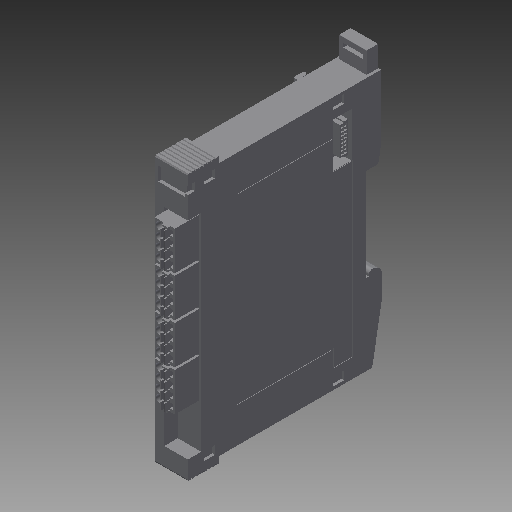
# Autodesk Inventor part: 178772
Saved by Autodesk Inventor 2019.3 (Build 233278000, 278)
## iProperties
Category: PARTsolutions
Company: MOELLER
Created: 2018-10-25
Part Number: 178772
Material: Generic
Catalog Web Link: www.cadenas.de
Description: I/O Modules-
Vendor: MOELLER
Document SubType Name: Modeling
Designer: psadmin
Manufacturer: MOELLER
Mass: 87.1869 g
Surface Area: 238.009 cm^2
Volume: 87.1869 cm^3
Density: 1 g/cm^3
Appearance: PSOLRGB-175-175-175
PSOL_IDENT_0: {$CADENAS_DATA\23d-libs\moeller\1589\1737\1739\1743\1744.prj},170 {VTYP=3D},{NB=178772},{LINA=178772
PSOL_IDENT_1: },{NN=I/O Modules},{DATE=04.10.2018 12:16:38},{GEOMDATE=04.10.2018 08:29:25},{VERSION=v181004082925}
PSOL_IDENT_2: ,{LINEID=10},{WBVAR=},{WBNUMERIC=}  {NB=178772},{LINA=178772},{KT=DUMMY},{PFOTO=2723pic-251.jpg},{PL
PSOL_IDENT_3: ID=178772},{DATA_SHEET=Data sheet},{MANUTYPEDESC=XN-322-4AI-PTNI},{DESCSHORT=Analog input module; 4
PSOL_IDENT_4: analog inputs; Pt/Ni/KTY/R with 2-wire or 3-wire connection},{DESCLONG=Analog input module for four
PSOL_IDENT_5: Pt100/Pt1000/Ni100/Ni1000/KTYxx/R resistance inputs with 2-wire and 3-wire configurations},{EAN=7640
PSOL_IDENT_6: 130098367},{ECLASS_8_1=27-24-26-01},{PACKAGED_WEIGHT=0.056},{DATA_SHEET_=http://datasheet.moeller.ne
PSOL_IDENT_7: t/datasheet.php?model=178772&locale=en_GB},{DATA_SHEET_ENG=http://datasheet.moeller.net/datasheet.ph
PSOL_IDENT_8: p?model=178772&locale=en_GB},{DATA_SHEET_DEU=http://datasheet.moeller.net/datasheet.php?model=178772
PSOL_IDENT_9: &locale=de_DE}
NN: I/O Modules
NB: 178772
NBSYN: $PLID.
LINA: 178772
PFOTO: 2723pic-251.jpg
PLID: 178772
DATA_SHEET: Data sheet
MANUTYPEDESC: XN-322-4AI-PTNI
DESCSHORT: Analog input module; 4 analog inputs; Pt/Ni/KTY/R with 2-wire or 3-wire connection
DESCLONG: Analog input module for four Pt100/Pt1000/Ni100/Ni1000/KTYxx/R resistance inputs with 2-wire and 3-wire configurations
EAN: 7640130098367
ECLASS_8_1: 27-24-26-01
PACKAGED_WEIGHT: 0.056
SUPPLIER: MOELLER
ARTICLENO: 178772
BOMINFO: 178772
CREATOR: CADENAS GmbH
Title: 178772
Author: Cadenas PARTsolutions
Autodesk Inventor part; units mm, degrees
(part 1 of 2)
ref_plane "YZ Plane" through (0, 0, 0) normal (1, 0, 0) x (0, 1, 0)
ref_plane "XZ Plane" through (0, 0, 0) normal (0, 1, 0) x (-1, 0, 0)
ref_plane "XY Plane" through (0, 0, 0) normal (0, 0, 1) x (1, 0, 0)
sketch "Sketch_31" plane through (0, 0, 0) normal (1, 0, 0) x (0, 1, 0)
  line L0 (50.4, 37) -> (-50.4, 37)
  line L1 (-50.4, 37) -> (-50.9, 36.75)
  line L2 (-50.9, 36.75) -> (-50.9, 35.75)
  line L3 (-50.9, 35.75) -> (-50.4, 35.5)
  line L4 (-50.4, 35.5) -> (-50.9, 35.25)
  line L5 (-50.9, 35.25) -> (-50.9, 34.25)
  line L6 (-50.9, 34.25) -> (-50.4, 34)
  line L7 (-50.4, 34) -> (-50.9, 33.75)
  line L8 (-50.9, 33.75) -> (-50.9, 32.75)
  line L9 (-50.9, 32.75) -> (-50.4, 32.5)
  line L10 (-50.4, 32.5) -> (-50.9, 32.25)
  line L11 (-50.9, 32.25) -> (-50.9, 31.25)
  line L12 (-50.9, 31.25) -> (-50.4, 31)
  line L13 (-50.4, 31) -> (-50.9, 30.75)
  line L14 (-50.9, 30.75) -> (-50.9, 29.75)
  line L15 (-50.9, 29.75) -> (-50.4, 29.5)
  line L16 (-50.4, 29.5) -> (-50.9, 29.25)
  line L17 (-50.9, 29.25) -> (-50.9, 28.25)
  line L18 (-50.9, 28.25) -> (-50.4, 28)
  line L19 (-50.4, 28) -> (-50.9, 27.75)
  line L20 (-50.9, 27.75) -> (-50.9, 26.75)
  line L21 (-50.9, 26.75) -> (-50.4, 26.5)
  line L22 (-50.4, 26.5) -> (-50.9, 26.25)
  line L23 (-50.9, 26.25) -> (-50.9, 25.25)
  line L24 (-50.9, 25.25) -> (-50.4, 25)
  line L25 (-50.4, 25) -> (-48.5, 25)
  line L26 (-48.5, 25) -> (-48.5, -32.7457)
  arc A0 (-48.5, -32.7457) -> (-47.6723, -33.7308) centre (-47.5, -32.7457) ccw
  line L27 (-47.6723, -33.7308) -> (-28.35, -37.11)
  line L28 (-28.35, -37.11) -> (-18.1454, -37.11)
  arc A1 (-18.1454, -37.11) -> (-17.2257, -36.6632) centre (-18.1454, -35.94) ccw
  line L29 (-17.2257, -36.6632) -> (-16.339, -35.5357)
  arc A2 (-16.339, -35.5357) -> (-16.3079, -35.4792) centre (-16.4962, -35.4121) ccw
  line L30 (-16.3079, -35.4792) -> (-15.785, -34.013)
  arc A3 (-15.785, -34.013) -> (-16.2215, -32.6577) centre (-16.887, -33.62) ccw
  line L31 (-16.2215, -32.6577) -> (-16.3517, -32.5677)
  arc A4 (-16.3517, -32.5677) -> (-17.0171, -32.36) centre (-17.0171, -33.53) ccw
  line L32 (-17.0171, -32.36) -> (-17.727, -32.36)
  line L33 (-17.727, -32.36) -> (-17.727, -31.25)
  line L34 (-17.727, -31.25) -> (17.833, -31.25)
  line L35 (17.833, -31.25) -> (17.833, -35.1079)
  arc A5 (17.833, -35.1079) -> (18.6743, -36.0952) centre (18.833, -35.1079) ccw
  line L36 (18.6743, -36.0952) -> (24.303, -37)
  line L37 (24.303, -37) -> (48.56, -37)
  line L38 (48.56, -37) -> (48.56, 25)
  line L39 (48.56, 25) -> (50.4, 25)
  line L40 (50.4, 25) -> (50.9, 25.25)
  line L41 (50.9, 25.25) -> (50.9, 26.25)
  line L42 (50.9, 26.25) -> (50.4, 26.5)
  line L43 (50.4, 26.5) -> (50.9, 26.75)
  line L44 (50.9, 26.75) -> (50.9, 27.75)
  line L45 (50.9, 27.75) -> (50.4, 28)
  line L46 (50.4, 28) -> (50.9, 28.25)
  line L47 (50.9, 28.25) -> (50.9, 29.25)
  line L48 (50.9, 29.25) -> (50.4, 29.5)
  line L49 (50.4, 29.5) -> (50.9, 29.75)
  line L50 (50.9, 29.75) -> (50.9, 30.75)
  line L51 (50.9, 30.75) -> (50.4, 31)
  line L52 (50.4, 31) -> (50.9, 31.25)
  line L53 (50.9, 31.25) -> (50.9, 32.25)
  line L54 (50.9, 32.25) -> (50.4, 32.5)
  line L55 (50.4, 32.5) -> (50.9, 32.75)
  line L56 (50.9, 32.75) -> (50.9, 33.75)
  line L57 (50.9, 33.75) -> (50.4, 34)
  line L58 (50.4, 34) -> (50.9, 34.25)
  line L59 (50.9, 34.25) -> (50.9, 35.25)
  line L60 (50.9, 35.25) -> (50.4, 35.5)
  line L61 (50.4, 35.5) -> (50.9, 35.75)
  line L62 (50.9, 35.75) -> (50.9, 36.75)
  line L63 (50.9, 36.75) -> (50.4, 37)
  constraints: 128 end point, 12 point on circle, 6 centre point
extrude "Extrusion1" add sketch "Sketch_31" along normal mid plane 12.5
sketch "Sketch_3" plane through (0, 0, 35.91) normal (0, 0, 1) x (1, 0, 0)
  line L0 (-2.75, 35.485) -> (-2.75, -43.665)
  line L1 (-2.75, -43.665) -> (6.25, -43.665)
  line L2 (6.25, -43.665) -> (6.25, 35.485)
  line L3 (6.25, 35.485) -> (-2.75, 35.485)
  constraints: 8 end point
extrude "Extrusion2" cut sketch "Sketch_3" along normal mid plane 8.12
sketch "Sketch_4" plane through (0, -4.03, 35.91) normal (0, 1, 0) x (1, 0, 0)
  line L0 (-2.242, 6.138) -> (-2.242, -5.332)
  line L1 (-2.242, -5.332) -> (5.508, -5.332)
  line L2 (5.508, -5.332) -> (5.508, 6.138)
  line L3 (5.508, 6.138) -> (-2.242, 6.138)
  constraints: 8 end point
extrude "Extrusion3" add sketch "Sketch_4" along normal mid plane 77.15
sketch "Sketch_7" plane through (0, 0, 35.91) normal (0, 0, 1) x (1, 0, 0)
  line L0 (-5.1, 48.02) -> (-5.1, 42.82)
  line L1 (-5.1, 42.82) -> (5.1, 42.82)
  line L2 (5.1, 42.82) -> (5.1, 43.92)
  line L3 (5.1, 43.92) -> (7.9, 43.92)
  line L4 (7.9, 43.92) -> (7.9, 46.92)
  line L5 (7.9, 46.92) -> (5.1, 46.92)
  line L6 (5.1, 46.92) -> (5.1, 48.02)
  line L7 (5.1, 48.02) -> (-5.1, 48.02)
  constraints: 16 end point
extrude "Extrusion4" cut sketch "Sketch_7" along normal mid plane 3.2
sketch "Sketch_8" plane through (0, 0, 35.91) normal (0, 0, 1) x (1, 0, 0)
  line L0 (-5, 47.92) -> (-5, 42.92)
  line L1 (-5, 42.92) -> (5, 42.92)
  line L2 (5, 42.92) -> (5, 47.92)
  line L3 (5, 47.92) -> (-5, 47.92)
  constraints: 8 end point
extrude "Extrusion5" add sketch "Sketch_8" against normal blind 2
sketch "Sketch_20" plane through (0, 0, 41.242) normal (0, 0, 1) x (1, 0, 0)
  line L0 (-2.165, -42.605) -> (2.835, -42.605)
  line L1 (2.835, -42.605) -> (2.835, 34.545)
  line L2 (2.835, 34.545) -> (-2.165, 34.545)
  line L3 (-2.165, 34.545) -> (-2.165, -42.605)
  constraints: 8 end point
sketch "Sketch_21" plane through (0, 0, 41.242) normal (0, 0, 1) x (1, 0, 0)
  line L0 (-2.165, -42.605) -> (2.835, -42.605)
  line L1 (2.835, -42.605) -> (2.835, 34.545)
  line L2 (2.835, 34.545) -> (-2.165, 34.545)
  line L3 (-2.165, 34.545) -> (-2.165, -42.605)
  circle A0 centre (-0.2, 32.542) radius 1.5
  circle A1 centre (-0.2, 29.042) radius 1.5
  circle A2 centre (-0.2, 25.542) radius 1.5
  circle A3 centre (-0.2, 22.042) radius 1.5
  circle A4 centre (-0.2, 16.942) radius 1.5
  circle A5 centre (-0.2, 13.442) radius 1.5
  circle A6 centre (-0.2, 9.942) radius 1.5
  circle A7 centre (-0.2, 6.442) radius 1.5
  circle A8 centre (-0.2, 1.342) radius 1.5
  circle A9 centre (-0.2, -2.158) radius 1.5
  circle A10 centre (-0.2, -5.658) radius 1.5
  circle A11 centre (-0.2, -9.158) radius 1.5
  circle A12 centre (-0.2, -14.258) radius 1.5
  circle A13 centre (-0.2, -17.758) radius 1.5
  circle A14 centre (-0.2, -21.258) radius 1.5
  circle A15 centre (-0.2, -24.758) radius 1.5
  circle A16 centre (-0.2, -29.858) radius 1.5
  circle A17 centre (-0.2, -33.358) radius 1.5
  circle A18 centre (-0.2, -36.858) radius 1.5
  circle A19 centre (-0.2, -40.358) radius 1.5
  constraints: 20 centre point, 8 end point
extrude "Extrusion6" cut sketch "Sketch_20" along normal mid plane 6.6
extrude "Extrusion7" add sketch "Sketch_21" against normal blind 3.3
sketch "Sketch_10" plane through (0, 0, 41.242) normal (0, 0, 1) x (1, 0, 0)
  line L0 (1.508, -42.605) -> (5.508, -42.605)
  line L1 (5.508, -42.605) -> (5.508, 34.545)
  line L2 (5.508, 34.545) -> (1.508, 34.545)
  line L3 (1.508, 34.545) -> (1.508, -42.605)
  constraints: 8 end point
sketch "Sketch_11" plane through (0, 0, 41.242) normal (0, 0, 1) x (1, 0, 0)
  line L0 (1.508, -42.605) -> (5.508, -42.605)
  line L1 (5.508, -42.605) -> (5.508, 34.545)
  line L2 (5.508, 34.545) -> (1.508, 34.545)
  line L3 (1.508, 34.545) -> (1.508, -42.605)
  line L4 (3.55, 31.392) -> (4.6, 31.392)
  arc A0 (4.6, 31.392) -> (4.9, 31.692) centre (4.6, 31.692) ccw
  line L5 (4.9, 31.692) -> (4.9, 33.142)
  arc A1 (4.9, 33.142) -> (4.6, 33.442) centre (4.6, 33.142) ccw
  line L6 (4.6, 33.442) -> (3.55, 33.442)
  line L7 (3.55, 33.442) -> (3.55, 31.392)
  line L8 (3.55, 27.892) -> (4.6, 27.892)
  arc A2 (4.6, 27.892) -> (4.9, 28.192) centre (4.6, 28.192) ccw
  line L9 (4.9, 28.192) -> (4.9, 29.642)
  arc A3 (4.9, 29.642) -> (4.6, 29.942) centre (4.6, 29.642) ccw
  line L10 (4.6, 29.942) -> (3.55, 29.942)
  line L11 (3.55, 29.942) -> (3.55, 27.892)
  line L12 (3.55, 24.392) -> (4.6, 24.392)
  arc A4 (4.6, 24.392) -> (4.9, 24.692) centre (4.6, 24.692) ccw
  line L13 (4.9, 24.692) -> (4.9, 26.142)
  arc A5 (4.9, 26.142) -> (4.6, 26.442) centre (4.6, 26.142) ccw
  line L14 (4.6, 26.442) -> (3.55, 26.442)
  line L15 (3.55, 26.442) -> (3.55, 24.392)
  line L16 (3.55, 20.892) -> (4.6, 20.892)
  arc A6 (4.6, 20.892) -> (4.9, 21.192) centre (4.6, 21.192) ccw
  line L17 (4.9, 21.192) -> (4.9, 22.642)
  arc A7 (4.9, 22.642) -> (4.6, 22.942) centre (4.6, 22.642) ccw
  line L18 (4.6, 22.942) -> (3.55, 22.942)
  line L19 (3.55, 22.942) -> (3.55, 20.892)
  line L20 (3.55, 15.792) -> (4.6, 15.792)
  arc A8 (4.6, 15.792) -> (4.9, 16.092) centre (4.6, 16.092) ccw
  line L21 (4.9, 16.092) -> (4.9, 17.542)
  arc A9 (4.9, 17.542) -> (4.6, 17.842) centre (4.6, 17.542) ccw
  line L22 (4.6, 17.842) -> (3.55, 17.842)
  line L23 (3.55, 17.842) -> (3.55, 15.792)
  line L24 (3.55, 12.292) -> (4.6, 12.292)
  arc A10 (4.6, 12.292) -> (4.9, 12.592) centre (4.6, 12.592) ccw
  line L25 (4.9, 12.592) -> (4.9, 14.042)
  arc A11 (4.9, 14.042) -> (4.6, 14.342) centre (4.6, 14.042) ccw
  line L26 (4.6, 14.342) -> (3.55, 14.342)
  line L27 (3.55, 14.342) -> (3.55, 12.292)
  line L28 (3.55, 8.792) -> (4.6, 8.792)
  arc A12 (4.6, 8.792) -> (4.9, 9.092) centre (4.6, 9.092) ccw
  line L29 (4.9, 9.092) -> (4.9, 10.542)
  arc A13 (4.9, 10.542) -> (4.6, 10.842) centre (4.6, 10.542) ccw
  line L30 (4.6, 10.842) -> (3.55, 10.842)
  line L31 (3.55, 10.842) -> (3.55, 8.792)
  line L32 (3.55, 5.292) -> (4.6, 5.292)
  arc A14 (4.6, 5.292) -> (4.9, 5.592) centre (4.6, 5.592) ccw
  line L33 (4.9, 5.592) -> (4.9, 7.042)
  arc A15 (4.9, 7.042) -> (4.6, 7.342) centre (4.6, 7.042) ccw
  line L34 (4.6, 7.342) -> (3.55, 7.342)
  line L35 (3.55, 7.342) -> (3.55, 5.292)
  line L36 (3.55, 0.192) -> (4.6, 0.192)
  arc A16 (4.6, 0.192) -> (4.9, 0.492) centre (4.6, 0.492) ccw
  line L37 (4.9, 0.492) -> (4.9, 1.942)
  arc A17 (4.9, 1.942) -> (4.6, 2.242) centre (4.6, 1.942) ccw
  line L38 (4.6, 2.242) -> (3.55, 2.242)
  line L39 (3.55, 2.242) -> (3.55, 0.192)
  line L40 (3.55, -3.308) -> (4.6, -3.308)
  arc A18 (4.6, -3.308) -> (4.9, -3.008) centre (4.6, -3.008) ccw
  line L41 (4.9, -3.008) -> (4.9, -1.558)
  arc A19 (4.9, -1.558) -> (4.6, -1.258) centre (4.6, -1.558) ccw
  line L42 (4.6, -1.258) -> (3.55, -1.258)
  line L43 (3.55, -1.258) -> (3.55, -3.308)
  line L44 (3.55, -6.808) -> (4.6, -6.808)
  arc A20 (4.6, -6.808) -> (4.9, -6.508) centre (4.6, -6.508) ccw
  line L45 (4.9, -6.508) -> (4.9, -5.058)
  arc A21 (4.9, -5.058) -> (4.6, -4.758) centre (4.6, -5.058) ccw
  line L46 (4.6, -4.758) -> (3.55, -4.758)
  line L47 (3.55, -4.758) -> (3.55, -6.808)
  line L48 (3.55, -10.308) -> (4.6, -10.308)
  arc A22 (4.6, -10.308) -> (4.9, -10.008) centre (4.6, -10.008) ccw
  line L49 (4.9, -10.008) -> (4.9, -8.558)
  arc A23 (4.9, -8.558) -> (4.6, -8.258) centre (4.6, -8.558) ccw
  line L50 (4.6, -8.258) -> (3.55, -8.258)
  line L51 (3.55, -8.258) -> (3.55, -10.308)
  line L52 (3.55, -15.408) -> (4.6, -15.408)
  arc A24 (4.6, -15.408) -> (4.9, -15.108) centre (4.6, -15.108) ccw
  line L53 (4.9, -15.108) -> (4.9, -13.658)
  arc A25 (4.9, -13.658) -> (4.6, -13.358) centre (4.6, -13.658) ccw
  line L54 (4.6, -13.358) -> (3.55, -13.358)
  line L55 (3.55, -13.358) -> (3.55, -15.408)
  line L56 (3.55, -18.908) -> (4.6, -18.908)
  arc A26 (4.6, -18.908) -> (4.9, -18.608) centre (4.6, -18.608) ccw
  line L57 (4.9, -18.608) -> (4.9, -17.158)
  arc A27 (4.9, -17.158) -> (4.6, -16.858) centre (4.6, -17.158) ccw
  line L58 (4.6, -16.858) -> (3.55, -16.858)
  line L59 (3.55, -16.858) -> (3.55, -18.908)
  line L60 (3.55, -22.408) -> (4.6, -22.408)
  arc A28 (4.6, -22.408) -> (4.9, -22.108) centre (4.6, -22.108) ccw
  line L61 (4.9, -22.108) -> (4.9, -20.658)
  arc A29 (4.9, -20.658) -> (4.6, -20.358) centre (4.6, -20.658) ccw
  line L62 (4.6, -20.358) -> (3.55, -20.358)
  line L63 (3.55, -20.358) -> (3.55, -22.408)
  line L64 (3.55, -25.908) -> (4.6, -25.908)
  arc A30 (4.6, -25.908) -> (4.9, -25.608) centre (4.6, -25.608) ccw
  line L65 (4.9, -25.608) -> (4.9, -24.158)
  arc A31 (4.9, -24.158) -> (4.6, -23.858) centre (4.6, -24.158) ccw
  line L66 (4.6, -23.858) -> (3.55, -23.858)
  line L67 (3.55, -23.858) -> (3.55, -25.908)
  line L68 (3.55, -31.008) -> (4.6, -31.008)
  arc A32 (4.6, -31.008) -> (4.9, -30.708) centre (4.6, -30.708) ccw
  line L69 (4.9, -30.708) -> (4.9, -29.258)
  arc A33 (4.9, -29.258) -> (4.6, -28.958) centre (4.6, -29.258) ccw
  line L70 (4.6, -28.958) -> (3.55, -28.958)
  line L71 (3.55, -28.958) -> (3.55, -31.008)
  line L72 (3.55, -34.508) -> (4.6, -34.508)
  arc A34 (4.6, -34.508) -> (4.9, -34.208) centre (4.6, -34.208) ccw
  line L73 (4.9, -34.208) -> (4.9, -32.758)
  arc A35 (4.9, -32.758) -> (4.6, -32.458) centre (4.6, -32.758) ccw
  line L74 (4.6, -32.458) -> (3.55, -32.458)
  line L75 (3.55, -32.458) -> (3.55, -34.508)
  line L76 (3.55, -38.008) -> (4.6, -38.008)
  arc A36 (4.6, -38.008) -> (4.9, -37.708) centre (4.6, -37.708) ccw
  line L77 (4.9, -37.708) -> (4.9, -36.258)
  arc A37 (4.9, -36.258) -> (4.6, -35.958) centre (4.6, -36.258) ccw
  line L78 (4.6, -35.958) -> (3.55, -35.958)
  line L79 (3.55, -35.958) -> (3.55, -38.008)
  line L80 (3.55, -41.508) -> (4.6, -41.508)
  arc A38 (4.6, -41.508) -> (4.9, -41.208) centre (4.6, -41.208) ccw
  line L81 (4.9, -41.208) -> (4.9, -39.758)
  arc A39 (4.9, -39.758) -> (4.6, -39.458) centre (4.6, -39.758) ccw
  line L82 (4.6, -39.458) -> (3.55, -39.458)
  line L83 (3.55, -39.458) -> (3.55, -41.508)
  constraints: 168 end point, 80 point on circle, 40 centre point
extrude "Extrusion8" cut sketch "Sketch_10" along normal mid plane 8
extrude "Extrusion9" add sketch "Sketch_11" against normal blind 4
sketch "Sketch_22" plane through (0, -4.03, 35.91) normal (0, 1, 0) x (1, 0, 0)
  line L0 (1.065, -5.332) -> (1.5846, -6.232)
  arc A0 (1.5846, -6.232) -> (1.7578, -6.332) centre (1.7578, -6.132) ccw
  line L1 (1.7578, -6.332) -> (3.658, -6.332)
  arc A1 (3.658, -6.332) -> (3.858, -6.132) centre (3.658, -6.132) ccw
  line L2 (3.858, -6.132) -> (3.858, -5.332)
  line L3 (3.858, -5.332) -> (1.065, -5.332)
  constraints: 8 end point, 4 point on circle, 2 centre point
extrude "Extrusion10" add sketch "Sketch_22" along normal mid plane 77.15
sketch "Sketch_9" plane through (0, 0, 0) normal (1, 0, 0) x (0, 1, 0)
  line L0 (33.95, 46.242) -> (-42, 46.242)
  line L1 (-42, 46.242) -> (-42, 41.242)
  line L2 (-42, 41.242) -> (-38.95, 41.242)
  line L3 (-38.95, 41.242) -> (-38.95, 44.242)
  line L4 (-38.95, 44.242) -> (-38.5, 44.242)
  line L5 (-38.5, 44.242) -> (-38.5, 41.242)
  line L6 (-38.5, 41.242) -> (-35.45, 41.242)
  line L7 (-35.45, 41.242) -> (-35.45, 44.242)
  line L8 (-35.45, 44.242) -> (-35, 44.242)
  line L9 (-35, 44.242) -> (-35, 41.242)
  line L10 (-35, 41.242) -> (-31.95, 41.242)
  line L11 (-31.95, 41.242) -> (-31.95, 44.242)
  line L12 (-31.95, 44.242) -> (-31.5, 44.242)
  line L13 (-31.5, 44.242) -> (-31.5, 41.242)
  line L14 (-31.5, 41.242) -> (-28.45, 41.242)
  line L15 (-28.45, 41.242) -> (-28.45, 44.242)
  line L16 (-28.45, 44.242) -> (-26.4, 44.242)
  line L17 (-26.4, 44.242) -> (-26.4, 41.242)
  line L18 (-26.4, 41.242) -> (-23.35, 41.242)
  line L19 (-23.35, 41.242) -> (-23.35, 44.242)
  line L20 (-23.35, 44.242) -> (-22.9, 44.242)
  line L21 (-22.9, 44.242) -> (-22.9, 41.242)
  line L22 (-22.9, 41.242) -> (-19.85, 41.242)
  line L23 (-19.85, 41.242) -> (-19.85, 44.242)
  line L24 (-19.85, 44.242) -> (-19.4, 44.242)
  line L25 (-19.4, 44.242) -> (-19.4, 41.242)
  line L26 (-19.4, 41.242) -> (-16.35, 41.242)
  line L27 (-16.35, 41.242) -> (-16.35, 44.242)
  line L28 (-16.35, 44.242) -> (-15.9, 44.242)
  line L29 (-15.9, 44.242) -> (-15.9, 41.242)
  line L30 (-15.9, 41.242) -> (-12.85, 41.242)
  line L31 (-12.85, 41.242) -> (-12.85, 44.242)
  line L32 (-12.85, 44.242) -> (-10.8, 44.242)
  line L33 (-10.8, 44.242) -> (-10.8, 41.242)
  line L34 (-10.8, 41.242) -> (-7.75, 41.242)
  line L35 (-7.75, 41.242) -> (-7.75, 44.242)
  line L36 (-7.75, 44.242) -> (-7.3, 44.242)
  line L37 (-7.3, 44.242) -> (-7.3, 41.242)
  line L38 (-7.3, 41.242) -> (-4.25, 41.242)
  line L39 (-4.25, 41.242) -> (-4.25, 44.242)
  line L40 (-4.25, 44.242) -> (-3.8, 44.242)
  line L41 (-3.8, 44.242) -> (-3.8, 41.242)
  line L42 (-3.8, 41.242) -> (-0.75, 41.242)
  line L43 (-0.75, 41.242) -> (-0.75, 44.242)
  line L44 (-0.75, 44.242) -> (-0.3, 44.242)
  line L45 (-0.3, 44.242) -> (-0.3, 41.242)
  line L46 (-0.3, 41.242) -> (2.75, 41.242)
  line L47 (2.75, 41.242) -> (2.75, 44.242)
  line L48 (2.75, 44.242) -> (4.8, 44.242)
  line L49 (4.8, 44.242) -> (4.8, 41.242)
  line L50 (4.8, 41.242) -> (7.85, 41.242)
  line L51 (7.85, 41.242) -> (7.85, 44.242)
  line L52 (7.85, 44.242) -> (8.3, 44.242)
  line L53 (8.3, 44.242) -> (8.3, 41.242)
  line L54 (8.3, 41.242) -> (11.35, 41.242)
  line L55 (11.35, 41.242) -> (11.35, 44.242)
  line L56 (11.35, 44.242) -> (11.8, 44.242)
  line L57 (11.8, 44.242) -> (11.8, 41.242)
  line L58 (11.8, 41.242) -> (14.85, 41.242)
  line L59 (14.85, 41.242) -> (14.85, 44.242)
  line L60 (14.85, 44.242) -> (15.3, 44.242)
  line L61 (15.3, 44.242) -> (15.3, 41.242)
  line L62 (15.3, 41.242) -> (18.35, 41.242)
  line L63 (18.35, 41.242) -> (18.35, 44.242)
  line L64 (18.35, 44.242) -> (20.4, 44.242)
  line L65 (20.4, 44.242) -> (20.4, 41.242)
  line L66 (20.4, 41.242) -> (23.45, 41.242)
  line L67 (23.45, 41.242) -> (23.45, 44.242)
  line L68 (23.45, 44.242) -> (23.9, 44.242)
  line L69 (23.9, 44.242) -> (23.9, 41.242)
  line L70 (23.9, 41.242) -> (26.95, 41.242)
  line L71 (26.95, 41.242) -> (26.95, 44.242)
  line L72 (26.95, 44.242) -> (27.4, 44.242)
  line L73 (27.4, 44.242) -> (27.4, 41.242)
  line L74 (27.4, 41.242) -> (30.45, 41.242)
  line L75 (30.45, 41.242) -> (30.45, 44.242)
  line L76 (30.45, 44.242) -> (30.9, 44.242)
  line L77 (30.9, 44.242) -> (30.9, 41.242)
  line L78 (30.9, 41.242) -> (33.95, 41.242)
  line L79 (33.95, 41.242) -> (33.95, 46.242)
  constraints: 160 end point
extrude "Extrusion11" cut sketch "Sketch_9" along normal blind 10
sketch "Sketch_12" plane through (0, -5.74, 0) normal (0, 1, 0) x (1, 0, 0)
  arc A0 (1.85, -43.03) -> (2.2465, -43.067) centre (2.05, -43.03) ccw
  line L0 (2.2465, -43.067) -> (2.4052, -42.2245)
  arc A1 (2.9948, -42.2245) -> (2.4052, -42.2245) centre (2.7, -42.28) ccw
  line L1 (2.9948, -42.2245) -> (3.1535, -43.067)
  arc A2 (3.1535, -43.067) -> (3.55, -43.03) centre (3.35, -43.03) ccw
  line L2 (3.55, -43.03) -> (3.55, -40.23)
  line L3 (3.55, -40.23) -> (1.85, -40.23)
  line L4 (1.85, -40.23) -> (1.85, -43.03)
  constraints: 10 end point, 6 point on circle, 3 centre point
extrude "Extrusion12" add sketch "Sketch_12" along normal mid plane 2.85
sketch "Sketch_13" plane through (0, -9.24, 0) normal (0, 1, 0) x (1, 0, 0)
  arc A0 (1.85, -43.03) -> (2.2465, -43.067) centre (2.05, -43.03) ccw
  line L0 (2.2465, -43.067) -> (2.4052, -42.2245)
  arc A1 (2.9948, -42.2245) -> (2.4052, -42.2245) centre (2.7, -42.28) ccw
  line L1 (2.9948, -42.2245) -> (3.1535, -43.067)
  arc A2 (3.1535, -43.067) -> (3.55, -43.03) centre (3.35, -43.03) ccw
  line L2 (3.55, -43.03) -> (3.55, -40.23)
  line L3 (3.55, -40.23) -> (1.85, -40.23)
  line L4 (1.85, -40.23) -> (1.85, -43.03)
  constraints: 10 end point, 6 point on circle, 3 centre point
sketch "Sketch_14" plane through (0, -14.38, 0) normal (0, 1, 0) x (1, 0, 0)
  arc A0 (1.85, -43.03) -> (2.2465, -43.067) centre (2.05, -43.03) ccw
  line L0 (2.2465, -43.067) -> (2.4052, -42.2245)
  arc A1 (2.9948, -42.2245) -> (2.4052, -42.2245) centre (2.7, -42.28) ccw
  line L1 (2.9948, -42.2245) -> (3.1535, -43.067)
  arc A2 (3.1535, -43.067) -> (3.55, -43.03) centre (3.35, -43.03) ccw
  line L2 (3.55, -43.03) -> (3.55, -40.23)
  line L3 (3.55, -40.23) -> (1.85, -40.23)
  line L4 (1.85, -40.23) -> (1.85, -43.03)
  constraints: 10 end point, 6 point on circle, 3 centre point
extrude "Extrusion13" add sketch "Sketch_13" along normal mid plane 2.85
extrude "Extrusion14" add sketch "Sketch_14" along normal mid plane 2.85
sketch "Sketch_15" plane through (0, -17.88, 0) normal (0, 1, 0) x (1, 0, 0)
  arc A0 (1.85, -43.03) -> (2.2465, -43.067) centre (2.05, -43.03) ccw
  line L0 (2.2465, -43.067) -> (2.4052, -42.2245)
  arc A1 (2.9948, -42.2245) -> (2.4052, -42.2245) centre (2.7, -42.28) ccw
  line L1 (2.9948, -42.2245) -> (3.1535, -43.067)
  arc A2 (3.1535, -43.067) -> (3.55, -43.03) centre (3.35, -43.03) ccw
  line L2 (3.55, -43.03) -> (3.55, -40.23)
  line L3 (3.55, -40.23) -> (1.85, -40.23)
  line L4 (1.85, -40.23) -> (1.85, -43.03)
  constraints: 10 end point, 6 point on circle, 3 centre point
extrude "Extrusion15" add sketch "Sketch_15" along normal mid plane 2.85
sketch "Sketch_16" plane through (0, -21.38, 0) normal (0, 1, 0) x (1, 0, 0)
  arc A0 (1.85, -43.03) -> (2.2465, -43.067) centre (2.05, -43.03) ccw
  line L0 (2.2465, -43.067) -> (2.4052, -42.2245)
  arc A1 (2.9948, -42.2245) -> (2.4052, -42.2245) centre (2.7, -42.28) ccw
  line L1 (2.9948, -42.2245) -> (3.1535, -43.067)
  arc A2 (3.1535, -43.067) -> (3.55, -43.03) centre (3.35, -43.03) ccw
  line L2 (3.55, -43.03) -> (3.55, -40.23)
  line L3 (3.55, -40.23) -> (1.85, -40.23)
  line L4 (1.85, -40.23) -> (1.85, -43.03)
  constraints: 10 end point, 6 point on circle, 3 centre point
extrude "Extrusion16" add sketch "Sketch_16" along normal mid plane 2.85
sketch "Sketch_17" plane through (0, -24.88, 0) normal (0, 1, 0) x (1, 0, 0)
  arc A0 (1.85, -43.03) -> (2.2465, -43.067) centre (2.05, -43.03) ccw
  line L0 (2.2465, -43.067) -> (2.4052, -42.2245)
  arc A1 (2.9948, -42.2245) -> (2.4052, -42.2245) centre (2.7, -42.28) ccw
  line L1 (2.9948, -42.2245) -> (3.1535, -43.067)
  arc A2 (3.1535, -43.067) -> (3.55, -43.03) centre (3.35, -43.03) ccw
  line L2 (3.55, -43.03) -> (3.55, -40.23)
  line L3 (3.55, -40.23) -> (1.85, -40.23)
  line L4 (1.85, -40.23) -> (1.85, -43.03)
  constraints: 10 end point, 6 point on circle, 3 centre point
extrude "Extrusion17" add sketch "Sketch_17" along normal mid plane 2.85
sketch "Sketch_18" plane through (0, -30.02, 0) normal (0, 1, 0) x (1, 0, 0)
  arc A0 (1.85, -43.03) -> (2.2465, -43.067) centre (2.05, -43.03) ccw
  line L0 (2.2465, -43.067) -> (2.4052, -42.2245)
  arc A1 (2.9948, -42.2245) -> (2.4052, -42.2245) centre (2.7, -42.28) ccw
  line L1 (2.9948, -42.2245) -> (3.1535, -43.067)
  arc A2 (3.1535, -43.067) -> (3.55, -43.03) centre (3.35, -43.03) ccw
  line L2 (3.55, -43.03) -> (3.55, -40.23)
  line L3 (3.55, -40.23) -> (1.85, -40.23)
  line L4 (1.85, -40.23) -> (1.85, -43.03)
  constraints: 10 end point, 6 point on circle, 3 centre point
extrude "Extrusion18" add sketch "Sketch_18" along normal mid plane 2.85
sketch "Sketch_19" plane through (0, -33.52, 0) normal (0, 1, 0) x (1, 0, 0)
  arc A0 (1.85, -43.03) -> (2.2465, -43.067) centre (2.05, -43.03) ccw
  line L0 (2.2465, -43.067) -> (2.4052, -42.2245)
  arc A1 (2.9948, -42.2245) -> (2.4052, -42.2245) centre (2.7, -42.28) ccw
  line L1 (2.9948, -42.2245) -> (3.1535, -43.067)
  arc A2 (3.1535, -43.067) -> (3.55, -43.03) centre (3.35, -43.03) ccw
  line L2 (3.55, -43.03) -> (3.55, -40.23)
  line L3 (3.55, -40.23) -> (1.85, -40.23)
  line L4 (1.85, -40.23) -> (1.85, -43.03)
  constraints: 10 end point, 6 point on circle, 3 centre point
extrude "Extrusion19" add sketch "Sketch_19" along normal mid plane 2.85
sketch "Sketch_23" plane through (0, -37.02, 0) normal (0, 1, 0) x (1, 0, 0)
  arc A0 (1.85, -43.03) -> (2.2465, -43.067) centre (2.05, -43.03) ccw
  line L0 (2.2465, -43.067) -> (2.4052, -42.2245)
  arc A1 (2.9948, -42.2245) -> (2.4052, -42.2245) centre (2.7, -42.28) ccw
  line L1 (2.9948, -42.2245) -> (3.1535, -43.067)
  arc A2 (3.1535, -43.067) -> (3.55, -43.03) centre (3.35, -43.03) ccw
  line L2 (3.55, -43.03) -> (3.55, -40.23)
  line L3 (3.55, -40.23) -> (1.85, -40.23)
  line L4 (1.85, -40.23) -> (1.85, -43.03)
  constraints: 10 end point, 6 point on circle, 3 centre point
extrude "Extrusion20" add sketch "Sketch_23" along normal mid plane 2.85
sketch "Sketch_24" plane through (0, -40.52, 0) normal (0, 1, 0) x (1, 0, 0)
  arc A0 (1.85, -43.03) -> (2.2465, -43.067) centre (2.05, -43.03) ccw
  line L0 (2.2465, -43.067) -> (2.4052, -42.2245)
  arc A1 (2.9948, -42.2245) -> (2.4052, -42.2245) centre (2.7, -42.28) ccw
  line L1 (2.9948, -42.2245) -> (3.1535, -43.067)
  arc A2 (3.1535, -43.067) -> (3.55, -43.03) centre (3.35, -43.03) ccw
  line L2 (3.55, -43.03) -> (3.55, -40.23)
  line L3 (3.55, -40.23) -> (1.85, -40.23)
  line L4 (1.85, -40.23) -> (1.85, -43.03)
  constraints: 10 end point, 6 point on circle, 3 centre point
extrude "Extrusion21" add sketch "Sketch_24" along normal mid plane 2.85
sketch "Sketch_25" plane through (6.25, 0, 0) normal (1, 0, 0) x (0, 0, -1)
  line L0 (18.627, 41.18) -> (18.627, 23.92)
  line L1 (18.627, 23.92) -> (25.827, 23.92)
  line L2 (25.827, 23.92) -> (25.827, 41.18)
  line L3 (25.827, 41.18) -> (18.627, 41.18)
  constraints: 8 end point
extrude "Extrusion22" cut sketch "Sketch_25" against normal blind 4.8
sketch "Sketch_48" plane through (1.45, 0, 0) normal (1, 0, 0) x (0, 0, -1)
  line L0 (20.696, 38.547) -> (20.696, 27.637)
  line L1 (20.696, 27.637) -> (22.196, 27.637)
  line L2 (22.196, 27.637) -> (22.196, 27.137)
  line L3 (22.196, 27.137) -> (23.746, 27.137)
  line L4 (23.746, 27.137) -> (23.746, 39.047)
  line L5 (23.746, 39.047) -> (22.196, 39.047)
  line L6 (22.196, 39.047) -> (22.196, 38.547)
  line L7 (22.196, 38.547) -> (20.696, 38.547)
  constraints: 16 end point
extrude "Extrusion23" add sketch "Sketch_48" along normal blind 5.35
sketch "Sketch_49" plane through (6.25, 0, 0) normal (1, 0, 0) x (0, 0, -1)
  line L0 (21.08, 38.07) -> (21.08, 28.11)
  line L1 (21.08, 28.11) -> (23.35, 28.11)
  line L2 (23.35, 28.11) -> (23.35, 38.07)
  line L3 (23.35, 38.07) -> (21.08, 38.07)
  constraints: 8 end point
extrude "Extrusion24" cut sketch "Sketch_49" along normal blind 0.55
sketch "Sketch_50" plane through (6.25, 0, 0) normal (1, 0, 0) x (0, 0, -1)
  line L0 (21.08, 30.45) -> (22.08, 30.45)
  line L1 (22.08, 30.45) -> (22.08, 29.38)
  line L2 (22.08, 29.38) -> (21.08, 29.38)
  line L3 (21.08, 29.38) -> (21.08, 29.18)
  line L4 (21.08, 29.18) -> (22.08, 29.18)
  line L5 (22.08, 29.18) -> (22.08, 28.11)
  line L6 (22.08, 28.11) -> (22.35, 28.11)
  line L7 (22.35, 28.11) -> (22.35, 29.18)
  line L8 (22.35, 29.18) -> (23.35, 29.18)
  line L9 (23.35, 29.18) -> (23.35, 29.38)
  line L10 (23.35, 29.38) -> (22.35, 29.38)
  line L11 (22.35, 29.38) -> (22.35, 30.45)
  line L12 (22.35, 30.45) -> (23.35, 30.45)
  line L13 (23.35, 30.45) -> (23.35, 30.65)
  line L14 (23.35, 30.65) -> (22.35, 30.65)
  line L15 (22.35, 30.65) -> (22.35, 31.72)
  line L16 (22.35, 31.72) -> (23.35, 31.72)
  line L17 (23.35, 31.72) -> (23.35, 31.92)
  line L18 (23.35, 31.92) -> (22.35, 31.92)
  line L19 (22.35, 31.92) -> (22.35, 32.99)
  line L20 (22.35, 32.99) -> (23.35, 32.99)
  line L21 (23.35, 32.99) -> (23.35, 33.19)
  line L22 (23.35, 33.19) -> (22.35, 33.19)
  line L23 (22.35, 33.19) -> (22.35, 34.26)
  line L24 (22.35, 34.26) -> (23.35, 34.26)
  line L25 (23.35, 34.26) -> (23.35, 34.46)
  line L26 (23.35, 34.46) -> (22.35, 34.46)
  line L27 (22.35, 34.46) -> (22.35, 35.53)
  line L28 (22.35, 35.53) -> (23.35, 35.53)
  line L29 (23.35, 35.53) -> (23.35, 35.73)
  line L30 (23.35, 35.73) -> (22.35, 35.73)
  line L31 (22.35, 35.73) -> (22.35, 36.8)
  line L32 (22.35, 36.8) -> (23.35, 36.8)
  line L33 (23.35, 36.8) -> (23.35, 37)
  line L34 (23.35, 37) -> (22.35, 37)
  line L35 (22.35, 37) -> (22.35, 38.07)
  line L36 (22.35, 38.07) -> (22.08, 38.07)
  line L37 (22.08, 38.07) -> (22.08, 37)
  line L38 (22.08, 37) -> (21.08, 37)
  line L39 (21.08, 37) -> (21.08, 36.8)
  line L40 (21.08, 36.8) -> (22.08, 36.8)
  line L41 (22.08, 36.8) -> (22.08, 35.73)
  line L42 (22.08, 35.73) -> (21.08, 35.73)
  line L43 (21.08, 35.73) -> (21.08, 35.53)
  line L44 (21.08, 35.53) -> (22.08, 35.53)
  line L45 (22.08, 35.53) -> (22.08, 34.46)
  line L46 (22.08, 34.46) -> (21.08, 34.46)
  line L47 (21.08, 34.46) -> (21.08, 34.26)
  line L48 (21.08, 34.26) -> (22.08, 34.26)
  line L49 (22.08, 34.26) -> (22.08, 33.19)
  line L50 (22.08, 33.19) -> (21.08, 33.19)
  line L51 (21.08, 33.19) -> (21.08, 32.99)
  line L52 (21.08, 32.99) -> (22.08, 32.99)
  line L53 (22.08, 32.99) -> (22.08, 31.92)
  line L54 (22.08, 31.92) -> (21.08, 31.92)
  line L55 (21.08, 31.92) -> (21.08, 31.72)
  line L56 (21.08, 31.72) -> (22.08, 31.72)
  line L57 (22.08, 31.72) -> (22.08, 30.65)
  line L58 (22.08, 30.65) -> (21.08, 30.65)
  line L59 (21.08, 30.65) -> (21.08, 30.45)
  constraints: 120 end point
extrude "Extrusion25" add sketch "Sketch_50" along normal blind 0.55
sketch "Sketch_27" plane through (-6.25, 0, 0) normal (1, 0, 0) x (0, 0, -1)
  line L0 (18.627, 42.21) -> (18.627, 23.92)
  line L1 (18.627, 23.92) -> (25.827, 23.92)
  line L2 (25.827, 23.92) -> (25.827, 42.21)
  line L3 (25.827, 42.21) -> (18.627, 42.21)
  constraints: 8 end point
extrude "Extrusion26" cut sketch "Sketch_27" along normal blind 1
sketch "Sketch_51" plane through (-10, 0, 0) normal (1, 0, 0) x (0, 0, -1)
  line L0 (20.13, 39.55) -> (20.13, 26.64)
  line L1 (20.13, 26.64) -> (24.33, 26.64)
  line L2 (24.33, 26.64) -> (24.33, 39.55)
  line L3 (24.33, 39.55) -> (20.13, 39.55)
  constraints: 8 end point
extrude "Extrusion27" add sketch "Sketch_51" along normal blind 4.75
sketch "Sketch_52" plane through (-6.25, 0, 0) normal (1, 0, 0) x (0, 0, -1)
  line L0 (20.696, 38.547) -> (20.696, 27.637)
  line L1 (20.696, 27.637) -> (22.196, 27.637)
  line L2 (22.196, 27.637) -> (22.196, 27.137)
  line L3 (22.196, 27.137) -> (23.746, 27.137)
  line L4 (23.746, 27.137) -> (23.746, 39.047)
  line L5 (23.746, 39.047) -> (22.196, 39.047)
  line L6 (22.196, 39.047) -> (22.196, 38.547)
  line L7 (22.196, 38.547) -> (20.696, 38.547)
  line L8 (22.7, 37.88) -> (22.7, 37.2)
  line L9 (22.7, 37.2) -> (23, 37.2)
  line L10 (23, 37.2) -> (23, 37.88)
  line L11 (23, 37.88) -> (22.7, 37.88)
  line L12 (22.7, 36.61) -> (22.7, 35.93)
  line L13 (22.7, 35.93) -> (23, 35.93)
  line L14 (23, 35.93) -> (23, 36.61)
  line L15 (23, 36.61) -> (22.7, 36.61)
  line L16 (22.7, 35.34) -> (22.7, 34.66)
  line L17 (22.7, 34.66) -> (23, 34.66)
  line L18 (23, 34.66) -> (23, 35.34)
  line L19 (23, 35.34) -> (22.7, 35.34)
  line L20 (22.7, 34.07) -> (22.7, 33.39)
  line L21 (22.7, 33.39) -> (23, 33.39)
  line L22 (23, 33.39) -> (23, 34.07)
  line L23 (23, 34.07) -> (22.7, 34.07)
  line L24 (22.7, 32.8) -> (22.7, 32.12)
  line L25 (22.7, 32.12) -> (23, 32.12)
  line L26 (23, 32.12) -> (23, 32.8)
  line L27 (23, 32.8) -> (22.7, 32.8)
  line L28 (22.7, 31.53) -> (22.7, 30.85)
  line L29 (22.7, 30.85) -> (23, 30.85)
  line L30 (23, 30.85) -> (23, 31.53)
  line L31 (23, 31.53) -> (22.7, 31.53)
  line L32 (22.7, 30.26) -> (22.7, 29.58)
  line L33 (22.7, 29.58) -> (23, 29.58)
  line L34 (23, 29.58) -> (23, 30.26)
  line L35 (23, 30.26) -> (22.7, 30.26)
  line L36 (22.7, 28.99) -> (22.7, 28.31)
  line L37 (22.7, 28.31) -> (23, 28.31)
  line L38 (23, 28.31) -> (23, 28.99)
  line L39 (23, 28.99) -> (22.7, 28.99)
  line L40 (21.43, 37.88) -> (21.43, 37.2)
  line L41 (21.43, 37.2) -> (21.73, 37.2)
  line L42 (21.73, 37.2) -> (21.73, 37.88)
  line L43 (21.73, 37.88) -> (21.43, 37.88)
  line L44 (21.43, 36.61) -> (21.43, 35.93)
  line L45 (21.43, 35.93) -> (21.73, 35.93)
  line L46 (21.73, 35.93) -> (21.73, 36.61)
  line L47 (21.73, 36.61) -> (21.43, 36.61)
  line L48 (21.43, 35.34) -> (21.43, 34.66)
  line L49 (21.43, 34.66) -> (21.73, 34.66)
  line L50 (21.73, 34.66) -> (21.73, 35.34)
  line L51 (21.73, 35.34) -> (21.43, 35.34)
  line L52 (21.43, 34.07) -> (21.43, 33.39)
  line L53 (21.43, 33.39) -> (21.73, 33.39)
  line L54 (21.73, 33.39) -> (21.73, 34.07)
  line L55 (21.73, 34.07) -> (21.43, 34.07)
  line L56 (21.43, 32.8) -> (21.43, 32.12)
  line L57 (21.43, 32.12) -> (21.73, 32.12)
  line L58 (21.73, 32.12) -> (21.73, 32.8)
  line L59 (21.73, 32.8) -> (21.43, 32.8)
  line L60 (21.43, 31.53) -> (21.43, 30.85)
  line L61 (21.43, 30.85) -> (21.73, 30.85)
  line L62 (21.73, 30.85) -> (21.73, 31.53)
  line L63 (21.73, 31.53) -> (21.43, 31.53)
  line L64 (21.43, 30.26) -> (21.43, 29.58)
  line L65 (21.43, 29.58) -> (21.73, 29.58)
  line L66 (21.73, 29.58) -> (21.73, 30.26)
  line L67 (21.73, 30.26) -> (21.43, 30.26)
  line L68 (21.43, 28.99) -> (21.43, 28.31)
  line L69 (21.43, 28.31) -> (21.73, 28.31)
  line L70 (21.73, 28.31) -> (21.73, 28.99)
  line L71 (21.73, 28.99) -> (21.43, 28.99)
  constraints: 144 end point
extrude "Extrusion28" cut sketch "Sketch_52" against normal blind 5
sketch "Sketch_53" plane through (-10, 0, 0) normal (1, 0, 0) x (0, 0, -1)
  line L0 (20.696, 38.547) -> (20.696, 27.637)
  line L1 (20.696, 27.637) -> (22.196, 27.637)
  line L2 (22.196, 27.637) -> (22.196, 27.137)
  line L3 (22.196, 27.137) -> (23.746, 27.137)
  line L4 (23.746, 27.137) -> (23.746, 39.047)
  line L5 (23.746, 39.047) -> (22.196, 39.047)
  line L6 (22.196, 39.047) -> (22.196, 38.547)
  line L7 (22.196, 38.547) -> (20.696, 38.547)
  constraints: 16 end point
extrude "Extrusion29" cut sketch "Sketch_53" along normal blind 1
sketch "Sketch_28" plane through (-6.25, 0, 0) normal (1, 0, 0) x (0, 0, -1)
  line L0 (-18.013, -35.03) -> (18.427, -35.03)
  line L1 (18.427, -35.03) -> (18.427, -41.3)
  line L2 (18.427, -41.3) -> (26.027, -41.3)
  line L3 (26.027, -41.3) -> (26.027, 23.92)
  line L4 (26.027, 23.92) -> (18.634, 23.92)
  line L5 (18.634, 23.92) -> (18.634, 35.12)
  line L6 (18.634, 35.12) -> (-18.013, 35.12)
  line L7 (-18.013, 35.12) -> (-18.013, -35.03)
  line L8 (-17.613, 34.72) -> (-17.613, -34.63)
  line L9 (-17.613, -34.63) -> (18.827, -34.63)
  line L10 (18.827, -34.63) -> (18.827, -40.9)
  line L11 (18.827, -40.9) -> (25.627, -40.9)
  line L12 (25.627, -40.9) -> (25.627, 23.77)
  line L13 (25.627, 23.77) -> (18.484, 23.77)
  line L14 (18.484, 23.77) -> (18.484, 34.72)
  line L15 (18.484, 34.72) -> (-17.613, 34.72)
  constraints: 32 end point
extrude "Extrusion30" cut sketch "Sketch_28" along normal mid plane 0.4
sketch "Sketch_29" plane through (6.25, 0, 0) normal (1, 0, 0) x (0, 0, -1)
  line L0 (-18.013, -35.03) -> (18.427, -35.03)
  line L1 (18.427, -35.03) -> (18.427, -41.3)
  line L2 (18.427, -41.3) -> (26.027, -41.3)
  line L3 (26.027, -41.3) -> (26.027, 23.92)
  line L4 (26.027, 23.92) -> (18.634, 23.92)
  line L5 (18.634, 23.92) -> (18.634, 35.12)
  line L6 (18.634, 35.12) -> (-18.013, 35.12)
  line L7 (-18.013, 35.12) -> (-18.013, -35.03)
  line L8 (-17.613, 34.72) -> (-17.613, -34.63)
  line L9 (-17.613, -34.63) -> (18.827, -34.63)
  line L10 (18.827, -34.63) -> (18.827, -40.9)
  line L11 (18.827, -40.9) -> (25.627, -40.9)
  line L12 (25.627, -40.9) -> (25.627, 23.77)
  line L13 (25.627, 23.77) -> (18.484, 23.77)
  line L14 (18.484, 23.77) -> (18.484, 34.72)
  line L15 (18.484, 34.72) -> (-17.613, 34.72)
  constraints: 32 end point
extrude "Extrusion31" cut sketch "Sketch_29" along normal mid plane 0.4
sketch "Sketch_1" plane through (0, 0, 0) normal (0, 1, 0) x (-1, 0, 0)
  line L0 (3.8, -43.69) -> (3.8, -33.69)
  line L1 (3.8, -33.69) -> (-3.8, -33.69)
  line L2 (-3.8, -33.69) -> (-3.8, -43.69)
  line L3 (-3.8, -43.69) -> (3.8, -43.69)
  constraints: 8 end point
extrude "Extrusion32" cut sketch "Sketch_1" along normal blind 50
sketch "Sketch_30" plane through (0, 0, 0) normal (1, 0, 0) x (0, 1, 0)
  line L0 (19.44, -32.17) -> (19.0775, -32.311)
  arc A0 (19.0775, -32.311) -> (18.95, -32.4974) centre (19.15, -32.4974) ccw
  line L1 (18.95, -32.4974) -> (18.95, -33.5037)
  arc A1 (18.95, -33.5037) -> (19.2284, -34.206) centre (19.975, -33.5037) ccw
  line L2 (19.2284, -34.206) -> (21.4964, -36.6173)
  arc A2 (21.4964, -36.6173) -> (22.2431, -36.94) centre (22.2431, -35.915) ccw
  line L3 (22.2431, -36.94) -> (56.45, -36.94)
  arc A3 (56.45, -36.94) -> (56.65, -36.74) centre (56.45, -36.74) ccw
  line L4 (56.65, -36.74) -> (56.65, -32.6982)
  arc A4 (56.65, -32.6982) -> (56.4518, -32.4982) centre (56.45, -32.6982) ccw
  line L5 (56.4518, -32.4982) -> (19.44, -32.17)
  constraints: 12 end point, 10 point on circle, 5 centre point
extrude "Extrusion33" add sketch "Sketch_30" along normal mid plane 10.49
sketch "Sketch_32" plane through (0, 0, -37.94) normal (0, 0, 1) x (1, 0, 0)
  line L0 (-3.75, 54.61) -> (-3.75, 53.11)
  line L1 (-3.75, 53.11) -> (3.76, 53.11)
  line L2 (3.76, 53.11) -> (3.76, 54.61)
  line L3 (3.76, 54.61) -> (-3.75, 54.61)
  constraints: 8 end point
extrude "Extrusion34" cut sketch "Sketch_32" along normal blind 11
sketch "Sketch_33" plane through (0, 0, -36.94) normal (0, 0, 1) x (1, 0, 0)
  line L0 (-2.105, 51.54) -> (-2.105, 41.98)
  line L1 (-2.105, 41.98) -> (2.105, 41.98)
  line L2 (2.105, 41.98) -> (2.105, 51.54)
  line L3 (2.105, 51.54) -> (-2.105, 51.54)
  constraints: 8 end point
extrude "Extrusion35" cut sketch "Sketch_33" along normal blind 1
sketch "Sketch_34" plane through (0, 0, -36.94) normal (0, 0, 1) x (1, 0, 0)
  line L0 (-3.8, 40.15) -> (-3.8, 29.27)
  line L1 (-3.8, 29.27) -> (3.8, 29.27)
  line L2 (3.8, 29.27) -> (3.8, 40.15)
  line L3 (3.8, 40.15) -> (-3.8, 40.15)
  constraints: 8 end point
extrude "Extrusion36" cut sketch "Sketch_34" along normal blind 4.3
sketch "Sketch_35" plane through (0, 0, -36.94) normal (0, 0, 1) x (1, 0, 0)
  arc A0 (-1.2855, 38.0537) -> (-2.2935, 36.901) centre (-2.25, 37.88) ccw
  line L0 (-2.2935, 36.901) -> (3.8, 36.63)
  line L1 (3.8, 36.63) -> (3.8, 38.13)
  line L2 (3.8, 38.13) -> (-1.0788, 37.8894)
  arc A1 (-1.2855, 38.0537) -> (-1.0788, 37.8894) centre (-1.0887, 38.0892) ccw
  constraints: 6 end point, 4 point on circle, 2 centre point
extrude "Extrusion37" add sketch "Sketch_35" along normal blind 4.3
sketch "Sketch_36" plane through (0, 0, -36.94) normal (0, 0, 1) x (1, 0, 0)
  line L0 (-3.8, 32.63) -> (2.2935, 32.901)
  arc A0 (2.2935, 32.901) -> (1.2855, 34.0537) centre (2.25, 33.88) ccw
  arc A1 (1.0788, 33.8894) -> (1.2855, 34.0537) centre (1.0887, 34.0892) ccw
  line L1 (1.0788, 33.8894) -> (-3.8, 34.13)
  line L2 (-3.8, 34.13) -> (-3.8, 32.63)
  constraints: 6 end point, 4 point on circle, 2 centre point
extrude "Extrusion38" add sketch "Sketch_36" along normal blind 4.3
sketch "Sketch_37" plane through (0, 0, -36.94) normal (0, 0, 1) x (1, 0, 0)
  line L0 (-3.8, 40.15) -> (-3.8, 29.27)
  line L1 (-3.8, 29.27) -> (3.8, 29.27)
  line L2 (3.8, 29.27) -> (3.8, 40.15)
  line L3 (3.8, 40.15) -> (-3.8, 40.15)
  constraints: 8 end point
extrude "Extrusion39" cut sketch "Sketch_37" along normal blind 2.2
sketch "Sketch_38" plane through (0, 0, -36.94) normal (0, 0, 1) x (1, 0, 0)
  line L0 (-2.105, 27.61) -> (-2.105, 22.95)
  line L1 (-2.105, 22.95) -> (2.105, 22.95)
  line L2 (2.105, 22.95) -> (2.105, 27.61)
  line L3 (2.105, 27.61) -> (-2.105, 27.61)
  constraints: 8 end point
extrude "Extrusion40" cut sketch "Sketch_38" along normal mid plane 2
sketch "Sketch_2" plane through (0, -2.283, 0) normal (0, 1, 0) x (1, 0, 0)
  arc A0 (1.85, -43.03) -> (2.2465, -43.067) centre (2.05, -43.03) ccw
  line L0 (2.2465, -43.067) -> (2.4052, -42.2245)
  arc A1 (2.9948, -42.2245) -> (2.4052, -42.2245) centre (2.7, -42.28) ccw
  line L1 (2.9948, -42.2245) -> (3.1535, -43.067)
  arc A2 (3.1535, -43.067) -> (3.55, -43.03) centre (3.35, -43.03) ccw
  line L2 (3.55, -43.03) -> (3.55, -40.23)
  line L3 (3.55, -40.23) -> (1.85, -40.23)
  line L4 (1.85, -40.23) -> (1.85, -43.03)
  constraints: 10 end point, 6 point on circle, 3 centre point
extrude "Extrusion41" add sketch "Sketch_2" along normal mid plane 2.85
sketch "Sketch_39" plane through (0, 1.217, 0) normal (0, 1, 0) x (1, 0, 0)
  arc A0 (1.85, -43.03) -> (2.2465, -43.067) centre (2.05, -43.03) ccw
  line L0 (2.2465, -43.067) -> (2.4052, -42.2245)
  arc A1 (2.9948, -42.2245) -> (2.4052, -42.2245) centre (2.7, -42.28) ccw
  line L1 (2.9948, -42.2245) -> (3.1535, -43.067)
  arc A2 (3.1535, -43.067) -> (3.55, -43.03) centre (3.35, -43.03) ccw
  line L2 (3.55, -43.03) -> (3.55, -40.23)
  line L3 (3.55, -40.23) -> (1.85, -40.23)
  line L4 (1.85, -40.23) -> (1.85, -43.03)
  constraints: 10 end point, 6 point on circle, 3 centre point
extrude "Extrusion42" add sketch "Sketch_39" along normal mid plane 2.85
sketch "Sketch_40" plane through (0, 6.317, 0) normal (0, 1, 0) x (1, 0, 0)
  arc A0 (1.85, -43.03) -> (2.2465, -43.067) centre (2.05, -43.03) ccw
  line L0 (2.2465, -43.067) -> (2.4052, -42.2245)
  arc A1 (2.9948, -42.2245) -> (2.4052, -42.2245) centre (2.7, -42.28) ccw
  line L1 (2.9948, -42.2245) -> (3.1535, -43.067)
  arc A2 (3.1535, -43.067) -> (3.55, -43.03) centre (3.35, -43.03) ccw
  line L2 (3.55, -43.03) -> (3.55, -40.23)
  line L3 (3.55, -40.23) -> (1.85, -40.23)
  line L4 (1.85, -40.23) -> (1.85, -43.03)
  constraints: 10 end point, 6 point on circle, 3 centre point
extrude "Extrusion43" add sketch "Sketch_40" along normal mid plane 2.85
sketch "Sketch_41" plane through (0, 9.817, 0) normal (0, 1, 0) x (1, 0, 0)
  arc A0 (1.85, -43.03) -> (2.2465, -43.067) centre (2.05, -43.03) ccw
  line L0 (2.2465, -43.067) -> (2.4052, -42.2245)
  arc A1 (2.9948, -42.2245) -> (2.4052, -42.2245) centre (2.7, -42.28) ccw
  line L1 (2.9948, -42.2245) -> (3.1535, -43.067)
  arc A2 (3.1535, -43.067) -> (3.55, -43.03) centre (3.35, -43.03) ccw
  line L2 (3.55, -43.03) -> (3.55, -40.23)
  line L3 (3.55, -40.23) -> (1.85, -40.23)
  line L4 (1.85, -40.23) -> (1.85, -43.03)
  constraints: 10 end point, 6 point on circle, 3 centre point
extrude "Extrusion44" add sketch "Sketch_41" along normal mid plane 2.85
sketch "Sketch_42" plane through (0, 13.317, 0) normal (0, 1, 0) x (1, 0, 0)
  arc A0 (1.85, -43.03) -> (2.2465, -43.067) centre (2.05, -43.03) ccw
  line L0 (2.2465, -43.067) -> (2.4052, -42.2245)
  arc A1 (2.9948, -42.2245) -> (2.4052, -42.2245) centre (2.7, -42.28) ccw
  line L1 (2.9948, -42.2245) -> (3.1535, -43.067)
  arc A2 (3.1535, -43.067) -> (3.55, -43.03) centre (3.35, -43.03) ccw
  line L2 (3.55, -43.03) -> (3.55, -40.23)
  line L3 (3.55, -40.23) -> (1.85, -40.23)
  line L4 (1.85, -40.23) -> (1.85, -43.03)
  constraints: 10 end point, 6 point on circle, 3 centre point
extrude "Extrusion45" add sketch "Sketch_42" along normal mid plane 2.85
sketch "Sketch_43" plane through (0, 16.817, 0) normal (0, 1, 0) x (1, 0, 0)
  arc A0 (1.85, -43.03) -> (2.2465, -43.067) centre (2.05, -43.03) ccw
  line L0 (2.2465, -43.067) -> (2.4052, -42.2245)
  arc A1 (2.9948, -42.2245) -> (2.4052, -42.2245) centre (2.7, -42.28) ccw
  line L1 (2.9948, -42.2245) -> (3.1535, -43.067)
  arc A2 (3.1535, -43.067) -> (3.55, -43.03) centre (3.35, -43.03) ccw
  line L2 (3.55, -43.03) -> (3.55, -40.23)
  line L3 (3.55, -40.23) -> (1.85, -40.23)
  line L4 (1.85, -40.23) -> (1.85, -43.03)
  constraints: 10 end point, 6 point on circle, 3 centre point
extrude "Extrusion46" add sketch "Sketch_43" along normal mid plane 2.85
sketch "Sketch_44" plane through (0, 21.917, 0) normal (0, 1, 0) x (1, 0, 0)
  arc A0 (1.85, -43.03) -> (2.2465, -43.067) centre (2.05, -43.03) ccw
  line L0 (2.2465, -43.067) -> (2.4052, -42.2245)
  arc A1 (2.9948, -42.2245) -> (2.4052, -42.2245) centre (2.7, -42.28) ccw
  line L1 (2.9948, -42.2245) -> (3.1535, -43.067)
  arc A2 (3.1535, -43.067) -> (3.55, -43.03) centre (3.35, -43.03) ccw
  line L2 (3.55, -43.03) -> (3.55, -40.23)
  line L3 (3.55, -40.23) -> (1.85, -40.23)
  line L4 (1.85, -40.23) -> (1.85, -43.03)
  constraints: 10 end point, 6 point on circle, 3 centre point
extrude "Extrusion47" add sketch "Sketch_44" along normal mid plane 2.85
sketch "Sketch_45" plane through (0, 25.417, 0) normal (0, 1, 0) x (1, 0, 0)
  arc A0 (1.85, -43.03) -> (2.2465, -43.067) centre (2.05, -43.03) ccw
  line L0 (2.2465, -43.067) -> (2.4052, -42.2245)
  arc A1 (2.9948, -42.2245) -> (2.4052, -42.2245) centre (2.7, -42.28) ccw
  line L1 (2.9948, -42.2245) -> (3.1535, -43.067)
  arc A2 (3.1535, -43.067) -> (3.55, -43.03) centre (3.35, -43.03) ccw
  line L2 (3.55, -43.03) -> (3.55, -40.23)
  line L3 (3.55, -40.23) -> (1.85, -40.23)
  line L4 (1.85, -40.23) -> (1.85, -43.03)
  constraints: 10 end point, 6 point on circle, 3 centre point
extrude "Extrusion48" add sketch "Sketch_45" along normal mid plane 2.85
sketch "Sketch_46" plane through (0, 28.917, 0) normal (0, 1, 0) x (1, 0, 0)
  arc A0 (1.85, -43.03) -> (2.2465, -43.067) centre (2.05, -43.03) ccw
  line L0 (2.2465, -43.067) -> (2.4052, -42.2245)
  arc A1 (2.9948, -42.2245) -> (2.4052, -42.2245) centre (2.7, -42.28) ccw
  line L1 (2.9948, -42.2245) -> (3.1535, -43.067)
  arc A2 (3.1535, -43.067) -> (3.55, -43.03) centre (3.35, -43.03) ccw
  line L2 (3.55, -43.03) -> (3.55, -40.23)
  line L3 (3.55, -40.23) -> (1.85, -40.23)
  line L4 (1.85, -40.23) -> (1.85, -43.03)
  constraints: 10 end point, 6 point on circle, 3 centre point
extrude "Extrusion49" add sketch "Sketch_46" along normal mid plane 2.85
sketch "Sketch_47" plane through (0, 32.417, 0) normal (0, 1, 0) x (1, 0, 0)
  arc A0 (1.85, -43.03) -> (2.2465, -43.067) centre (2.05, -43.03) ccw
  line L0 (2.2465, -43.067) -> (2.4052, -42.2245)
  arc A1 (2.9948, -42.2245) -> (2.4052, -42.2245) centre (2.7, -42.28) ccw
  line L1 (2.9948, -42.2245) -> (3.1535, -43.067)
  arc A2 (3.1535, -43.067) -> (3.55, -43.03) centre (3.35, -43.03) ccw
  line L2 (3.55, -43.03) -> (3.55, -40.23)
  line L3 (3.55, -40.23) -> (1.85, -40.23)
  line L4 (1.85, -40.23) -> (1.85, -43.03)
  constraints: 10 end point, 6 point on circle, 3 centre point
extrude "Extrusion50" add sketch "Sketch_47" along normal mid plane 2.85
sketch "Sketch_60" plane through (6.25, 0, 0) normal (1, 0, 0) x (0, 0, -1)
  line L0 (18.67, 47.51) -> (18.67, 44.3)
  line L1 (18.67, 44.3) -> (22.88, 44.3)
  line L2 (22.88, 44.3) -> (22.88, 47.51)
  line L3 (22.88, 47.51) -> (18.67, 47.51)
  constraints: 8 end point
extrude "Extrusion51" cut sketch "Sketch_60" along normal mid plane 2
sketch "Sketch_61" plane through (6.25, 0, 0) normal (1, 0, 0) x (0, 0, -1)
  line L0 (-30.83, -44.09) -> (-30.83, -47.3)
  line L1 (-30.83, -47.3) -> (-26.62, -47.3)
  line L2 (-26.62, -47.3) -> (-26.62, -44.09)
  line L3 (-26.62, -44.09) -> (-30.83, -44.09)
  constraints: 8 end point
extrude "Extrusion52" cut sketch "Sketch_61" along normal mid plane 2
sketch "Sketch_54" plane through (0, -45.7, 0) normal (0, 1, 0) x (1, 0, 0)
  line L0 (-9.05, -27.23) -> (-9.05, -30.43)
  arc A0 (-9.05, -30.43) -> (-8.65, -30.83) centre (-8.65, -30.43) ccw
  line L1 (-8.65, -30.83) -> (-5.25, -30.83)
  line L2 (-5.25, -30.83) -> (-5.25, -28.83)
  line L3 (-5.25, -28.83) -> (-7.45, -28.83)
  line L4 (-7.45, -28.83) -> (-7.45, -27.83)
  line L5 (-7.45, -27.83) -> (-8.05, -26.83)
  line L6 (-8.05, -26.83) -> (-8.65, -26.83)
  arc A1 (-8.65, -26.83) -> (-9.05, -27.23) centre (-8.65, -27.23) ccw
  constraints: 14 end point, 4 point on circle, 2 centre point
sketch "Sketch_55" plane through (0, 45.9, 0) normal (0, 1, 0) x (1, 0, 0)
  line L0 (-9.05, -27.23) -> (-9.05, -30.43)
  arc A0 (-9.05, -30.43) -> (-8.65, -30.83) centre (-8.65, -30.43) ccw
  line L1 (-8.65, -30.83) -> (-5.25, -30.83)
  line L2 (-5.25, -30.83) -> (-5.25, -28.83)
  line L3 (-5.25, -28.83) -> (-7.45, -28.83)
  line L4 (-7.45, -28.83) -> (-7.45, -27.83)
  line L5 (-7.45, -27.83) -> (-8.05, -26.83)
  line L6 (-8.05, -26.83) -> (-8.65, -26.83)
  arc A1 (-8.65, -26.83) -> (-9.05, -27.23) centre (-8.65, -27.23) ccw
  constraints: 14 end point, 4 point on circle, 2 centre point